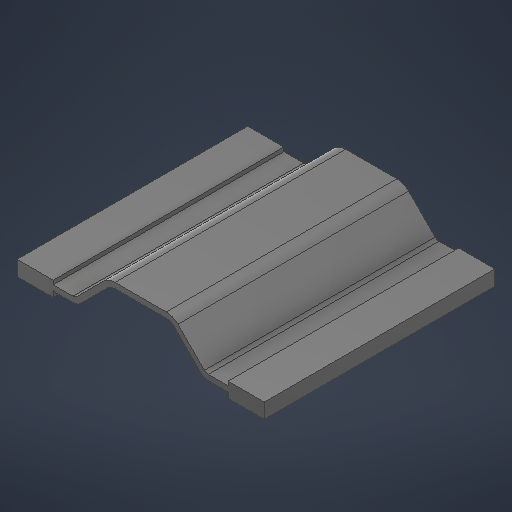
# Autodesk Inventor part: Monitor Base Slide v1.0
Saved by Autodesk Inventor 2027 (Build 310192060, 192F)
## iProperties
Created: 2026-05-19
Part Number: Monitor Base Slide v1.0
Material: Generic
Document SubType Name: Modeling
Designer: cheap
Density: 1 g/cm^3
Appearance: Default
Author: cheap
Autodesk Inventor part; units mm, degrees
ref_plane "YZ Plane" through (0, 0, 0) normal (1, 0, 0) x (0, 1, 0)
ref_plane "XZ Plane" through (0, 0, 0) normal (0, 1, 0) x (-1, 0, 0)
ref_plane "XY Plane" through (0, 0, 0) normal (0, 0, 1) x (1, 0, 0)
sketch "Sketch1" plane through (0, 0, 0) normal (0, 0, 1) x (1, 0, 0)
  line L0 (10.4513, 0) -> (16.1601, 0)
  line L1 (18.4051, 0.9299) -> (26.0858, 8.6106)
  line L2 (28.3309, 9.5406) -> (43.1193, 9.5406)
  line L3 (45.3644, 8.6106) -> (53.0451, 0.9299)
  line L4 (55.2901, 0) -> (60.9989, 0)
  arc A0 (16.1601, 0) -> (18.4051, 0.9299) centre (16.1601, 3.175) ccw
  arc A1 (28.3309, 9.5406) -> (26.0858, 8.6106) centre (28.3309, 6.3656) ccw
  arc A2 (45.3644, 8.6106) -> (43.1193, 9.5406) centre (43.1193, 6.3656) ccw
  arc A3 (53.0451, 0.9299) -> (55.2901, 0) centre (55.2901, 3.175) ccw
  line L5 (60.9989, 1.5875) -> (55.2901, 1.5875)
  arc A4 (54.1676, 2.0525) -> (55.2901, 1.5875) centre (55.2901, 3.175) ccw
  line L6 (54.1676, 2.0525) -> (46.4869, 9.7332)
  arc A5 (46.4869, 9.7332) -> (43.1193, 11.1281) centre (43.1193, 6.3656) ccw
  line L7 (43.1193, 11.1281) -> (28.3309, 11.1281)
  arc A6 (28.3309, 11.1281) -> (24.9633, 9.7332) centre (28.3309, 6.3656) ccw
  line L8 (24.9633, 9.7332) -> (17.2826, 2.0525)
  arc A7 (16.1601, 1.5875) -> (17.2826, 2.0525) centre (16.1601, 3.175) ccw
  line L9 (16.1601, 1.5875) -> (10.4513, 1.5875)
  line L10 (10.4513, 1.5875) -> (10.4513, 2.7388)
  line L11 (10.4513, 2.7388) -> (0, 2.7388)
  line L12 (0, 0) -> (0, 2.7388)
  line L13 (0, 0) -> (0, 0.5757)
  line L14 (60.9989, 1.5875) -> (60.9989, 2.7388)
  line L15 (60.9989, 2.7388) -> (71.4502, 2.7388)
  line L16 (71.4502, 0) -> (71.4502, 2.7388)
  line L17 (71.4502, 0) -> (71.4502, 0.5757)
  line L18 (10.4513, 0) -> (10.4513, -1.5875)
  line L19 (10.4513, -1.5875) -> (0, -1.5875)
  line L20 (0, -1.5875) -> (0, 0)
  line L21 (60.9989, 0) -> (60.9989, -1.5875)
  line L22 (60.9989, -1.5875) -> (71.4502, -1.5875)
  line L23 (71.4502, -1.5875) -> (71.4502, 0)
  point P0 (17.4752, 0)
  point P1 (53.975, 0)
  dimension "d6" = 135
  dimension "d7" = 135
  dimension "d9" = 3.175
  dimension "d10" = 1.5875
  dimension "d15" = 1.5875
  constraints: 48 end point, 16 point on circle, 8 centre point, 8 tangent, 6 perpendicular, 6 point on line, 3 equal radius, 2 parallel, 2 vertical, 1 horizontal, 6 other
  measures "d6" angle of L1 L2
  measures "d7" angle of L3 L2
  measures "d9" radius of A0
  measures "d10" distance between parallel lines of L1 L8
  measures "d15" distance of L4.end L21.end
extrude "Extrusion2" add sketch "Sketch1" along normal blind 66.675
body "Solid2"
